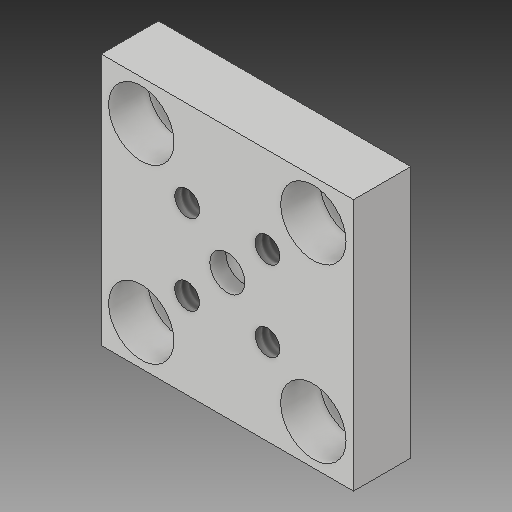
# Autodesk Inventor part: sample holder mount on PI_V_522_v2
Saved by Autodesk Inventor 2019 (Build 230136000, 136)
## iProperties
Created: 2018-07-23
Part Number: sample holder mount on PI_V_522_v2
Material: Generic
Document SubType Name: Sheet Metal
Designer: FiolkaLab
Density: 1 g/cm^3
Sheet Metal Rule: Default_mm
Appearance: Default
Author: FiolkaLab
Autodesk Inventor part; units mm, degrees
ref_plane "YZ Plane" through (0, 0, 0) normal (1, 0, 0) x (0, 1, 0)
ref_plane "XZ Plane" through (0, 0, 0) normal (0, 1, 0) x (-1, 0, 0)
ref_plane "XY Plane" through (0, 0, 0) normal (0, 0, 1) x (1, 0, 0)
sketch "Sketch1" plane through (0, 0, 0) normal (0, 0, 1) x (1, 0, 0)
  line L0 (0, 0) -> (22, 0)
  line L1 (22, 0) -> (22, 22)
  line L2 (22, 22) -> (0, 22)
  line L3 (0, 22) -> (0, 0)
  dimension "d0" = 22
  dimension "d1" = 22
  constraints: 8 end point, 2 parallel, 1 horizontal, 1 perpendicular
  measures "d0" distance of L1.end L2.end
  measures "d1" distance of L0.end L1.end
extrude "Extrusion1" add sketch "Sketch1" along normal blind 5
sketch "Sketch2" plane through (0, 0, 5) normal (0, 0, 1) x (1, 0, 0)
  circle A0 centre (3.5, 18.5) radius 1.5
  circle A1 centre (18.5, 18.5) radius 1.5
  line L0 (0, 22) -> (0, 0) projected
  line L1 (22, 22) -> (0, 22) projected
  circle A2 centre (3.5, 3.5) radius 1.5
  line L2 (0, 0) -> (22, 0) projected
  circle A3 centre (18.5, 3.5) radius 1.5
  line L3 (22, 0) -> (22, 22) projected
  dimension "d4" = 3
  dimension "d5" = 3
  dimension "d6" = 3.5
  dimension "d7" = 15
  dimension "d8" = 3.5
  dimension "d9" = 3.5
  dimension "d10" = 3
  dimension "d11" = 3.5
  dimension "d12" = 3.5
  dimension "d13" = 3
  dimension "d14" = 3.5
  dimension "d15" = 3.5
  constraints: 4 centre point
  measures "d4" diameter of A0
  measures "d5" diameter of A1
  measures "d6" distance from line of L0 A0.centre
  measures "d7" distance of A1.centre A0.centre
  measures "d8" distance from line of A1.centre L1
  measures "d9" distance from line of L1 A0.centre
  measures "d10" diameter of A2
  measures "d11" distance from line of L2 A2.centre
  measures "d12" distance from line of L0 A2.centre
  measures "d13" diameter of A3
  measures "d14" distance from line of L2 A3.centre
  measures "d15" distance from line of A3.centre L3
hole "Hole1" at (3.5, 18.5, 5) at (18.5, 18.5, 5) at (18.5, 3.5, 5) at (3.5, 3.5, 5) direction (0, 0, -1) diameter 3.2 end through all counterbore diameter 5.7 counterbore depth 3.4
sketch "Sketch3" plane through (0, 0, 5) normal (0, 0, 1) x (1, 0, 0)
  circle A0 centre (7.5, 7.5) radius 1.5
  line L0 (0, 22) -> (0, 0) projected
  line L1 (0, 0) -> (22, 0) projected
  circle A1 centre (7.5, 14.5) radius 1.5
  circle A2 centre (14.5, 7.5) radius 1.5
  circle A3 centre (14.5, 14.5) radius 1.5
  dimension "d23" = 3
  dimension "d24" = 7.5
  dimension "d25" = 7.5
  dimension "d33" = 3
  dimension "d34" = 3
  dimension "d35" = 3
  dimension "d36" = 7
  dimension "d37" = 7
  dimension "d38" = 7
  dimension "d39" = 0
  dimension "d40" = 7.5
  dimension "d41" = 7
  constraints: 4 centre point
  measures "d23" diameter of A0
  measures "d24" distance from line of L0 A0.centre
  measures "d25" distance from line of L1 A0.centre
  measures "d33" diameter of A1
  measures "d34" diameter of A2
  measures "d35" diameter of A3
  measures "d36" distance of A3.centre A2.centre
  measures "d37" distance of A3.centre A1.centre
  measures "d38" distance of A1.centre A0.centre
  measures "d39" horizontal distance of A1.centre A0.centre
  measures "d40" distance from line of L1 A2.centre
  measures "d41" distance of A0.centre A2.centre
hole "Hole2" at (7.5, 7.5, 5) at (7.5, 14.5, 5) at (14.5, 7.5, 5) at (14.5, 14.5, 5) direction (0, 0, -1) diameter 2.156 end through all thread size "4-40 UNC" class "2B" standard "ANSI Unified Screw Threads"
sketch "Sketch7" plane through (0, 0, 5) normal (0, 0, 1) x (1, 0, 0)
  circle A0 centre (11, 11) radius 1.5
  line L0 (22, 22) -> (0, 22) projected
  line L1 (22, 0) -> (22, 22) projected
  point P0 (0, 0)
  dimension "d64" = 3
  dimension "d65" = 11
  dimension "d66" = 11
  constraints: 1 centre point
  measures "d64" diameter of A0
  measures "d65" distance from line of L0 A0.centre
  measures "d66" distance from line of L1 A0.centre
hole "Hole5" at (11, 11, 5) direction (0, 0, -1) diameter 3.05 end through all
sketch "Sketch8" plane through (0, 0, 0) normal (0, 0, -1) x (-1, 0, 0)
  circle A0 centre (-11, 11) radius 1.525 projected
  circle A1 centre (-11, 11) radius 2.45
  point P0 (0, 0)
  dimension "d74" = 4.9
  constraints: 1 centre point, 1 coincident
  measures "d74" diameter of A1
hole "Hole6" at (11, 11, 0) direction (0, 0, 1) diameter 4.9 depth 3.05 tip angle 118
equation "\"d21\" = Thickness"
equation "\"d23\" = d35"
equation "\"d33\" = d35"
equation "\"d34\" = d35"
equation "\"d36\" = d38"
equation "\"d37\" = d38"
equation "\"d40\" = d25"
equation "\"BendRadius\" = Thickness"
equation "\"BendReliefWidth\" = Thickness"
equation "\"BendReliefDepth\" = 0.5 * Thickness"
equation "\"CornerReliefSize\" = 4 * Thickness"
equation "\"MinimumRemnant\" = 2 * Thickness"
equation "\"TransitionRadius\" = BendRadius"
equation "\"JacobiRadiusSize\" = BendRadius"
equation "\"GapSize\" = Thickness"
equation "\"Thickness\" = 0.5"
body "Solid1"
